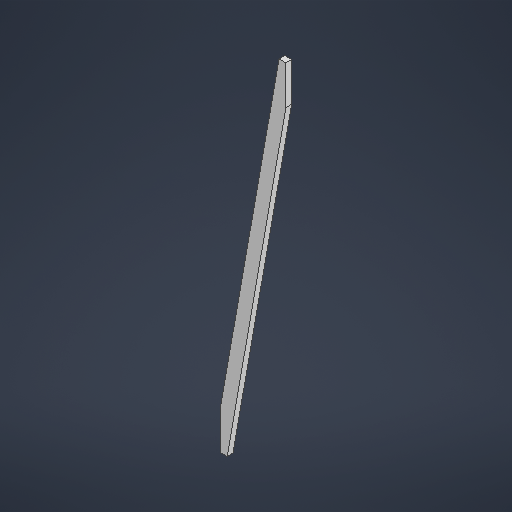
# Autodesk Inventor part: S_2x4x97.494
Saved by Autodesk Inventor 2026 (Build 300175000, 175)
## iProperties
Created: 2025-09-05
Part Number: S_2x4x97.494
Material: Generic
Document SubType Name: Modeling
Designer: trott
Density: 1 g/cm^3
Appearance: Default
Author: trott
Autodesk Inventor part; units mm, degrees
ref_plane "YZ Plane" through (0, 0, 0) normal (1, 0, 0) x (0, 1, 0)
ref_plane "XZ Plane" through (0, 0, 0) normal (0, 1, 0) x (-1, 0, 0)
ref_plane "XY Plane" through (0, 0, 0) normal (0, 0, 1) x (1, 0, 0)
sketch "Sketch1" plane through (0, 0, 0) normal (0, 0, 1) x (1, 0, 0)
  line L0 (215.9, -1219.2) -> (-215.9, -1219.2)
  line L1 (-215.9, -1219.2) -> (-215.9, 1219.2)
  line L2 (-215.9, 1219.2) -> (215.9, 1219.2)
  line L3 (215.9, 1219.2) -> (215.9, -1219.2)
  line L4 (215.9, -1219.2) -> (-215.9, 1219.2) construction
  line L5 (-215.9, -1219.2) -> (215.9, 1219.2) construction
  line L6 (215.9, 1219.2) -> (-215.9, -1219.2)
  line L7 (-172.131, -1226.9508) -> (-259.669, -1211.4492)
  line L8 (259.669, 1211.4492) -> (172.131, 1226.9508)
  line L9 (259.669, 1211.4492) -> (-172.131, -1226.9508)
  line L10 (-259.669, -1211.4492) -> (172.131, 1226.9508)
  point P0 (0, 0)
  point P1 (-170.7584, -1219.2)
  point P2 (215.9, 964.2829)
  point P3 (170.7584, 1219.2)
  point P4 (-215.9, -964.2829)
  dimension "d0" = 431.8
  dimension "d1" = 2438.4
  dimension "d2" = 88.9
  dimension "d3" = 88.9
  constraints: 22 end point, 4 midpoint, 3 parallel, 3 perpendicular, 1 horizontal
  measures "d0" distance of L1.end L2.end
  measures "d1" distance of L0.end L1.end
  measures "d2" distance of L7.start L7.end
  measures "d3" distance of L8.start L8.end
extrude "Extrusion1" add sketch "Sketch1" along normal blind 38.1 contours L0 L6 L3 L9 | L1 L10 L2 L6
body "Solid1"
